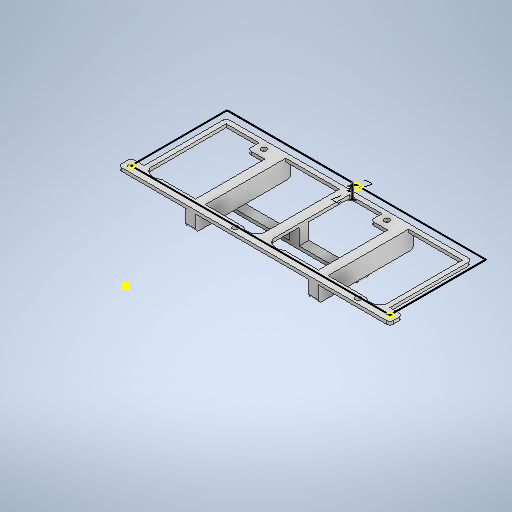
# Autodesk Inventor part: hackatonski skurwiel
Saved by Autodesk Inventor 2025.2 (Build 292293000, 293)
## iProperties
Created: 2026-03-22
Part Number: hackatonski skurwiel
Material: Ogólny
Document SubType Name: Modeling
Designer: janla
Density: 1 g/cm^3
Appearance: Domyślna
Author: janla
Autodesk Inventor part; units mm, degrees
ref_plane "YZ Plane" through (0, 0, 0) normal (1, 0, 0) x (0, 1, 0)
ref_plane "XZ Plane" through (0, 0, 0) normal (0, 1, 0) x (-1, 0, 0)
ref_plane "XY Plane" through (0, 0, 0) normal (0, 0, 1) x (1, 0, 0)
sketch "Szkic1" plane through (0, 0, 0) normal (0, 1, 0) x (-1, 0, 0)
  line L0 (-78.5676, -65.5638) -> (-27.7676, -65.5638)
  line L1 (-27.7676, -65.5638) -> (-27.7676, -111.2838)
  line L2 (-27.7676, -111.2838) -> (-78.5676, -111.2838)
  line L3 (-78.5676, -111.2838) -> (-78.5676, -65.5638)
  circle A0 centre (-78.5676, -65.5638) radius 1.65
  line L4 (-27.7676, -65.5638) -> (-27.7676, -116.3638)
  line L5 (-27.7676, -116.3638) -> (-45.5476, -116.3638)
  circle A1 centre (-45.5476, -116.3638) radius 1.65
  line L6 (-80.2176, -65.5638) -> (-90.2176, -65.5638)
  line L7 (-90.2176, -65.5638) -> (-90.2176, -68.5638)
  line L8 (-90.2176, -68.5638) -> (-90.2176, -62.5638)
  line L9 (-90.2176, -62.5638) -> (-20.2176, -62.5638)
  line L10 (-20.2176, -62.5638) -> (-20.2176, -68.5638)
  line L11 (-20.2176, -68.5638) -> (-90.2176, -68.5638)
  line L12 (-78.5676, -68.5638) -> (-90.2176, -68.5638)
  line L13 (-84.3926, -68.5638) -> (-84.3926, -73.5638)
  circle A2 centre (-84.3926, -73.5638) radius 6.35
  line L14 (-55.2176, -68.5638) -> (-55.2176, -111.2838)
  line L15 (-31.8676, -111.2838) -> (-31.8676, -65.5638)
  line L16 (-20.2176, -65.5638) -> (-20.2176, -68.5638)
  line L17 (-20.2176, -68.5638) -> (-20.2176, -62.5638)
  line L18 (-90.2176, -68.5638) -> (-20.2176, -68.5638)
  line L19 (-31.8676, -68.5638) -> (-20.2176, -68.5638)
  line L20 (-26.0426, -68.5638) -> (-26.0426, -73.5638)
  circle A3 centre (-26.0426, -73.5638) radius 6.35
  line L21 (-45.5476, -116.3638) -> (-40.5476, -116.3638)
  line L22 (-40.5476, -116.3638) -> (-40.5476, -121.3638)
  line L23 (-40.5476, -121.3638) -> (-50.5476, -121.3638)
  line L24 (-50.5476, -121.3638) -> (-50.5476, -111.3638)
  line L25 (-50.5476, -111.3638) -> (-40.5476, -111.3638)
  line L26 (-40.5476, -111.3638) -> (-40.5476, -121.3638)
  line L27 (-45.5476, -116.3638) -> (-54.0476, -116.3638)
  line L28 (-54.0476, -116.3638) -> (-51.0476, -116.3638)
  line L29 (-51.0476, -116.3638) -> (-51.0476, -68.5638)
  line L30 (-51.0476, -68.5638) -> (-54.0476, -68.5638)
  line L31 (-54.0476, -68.5638) -> (-54.0476, -116.3638)
  line L32 (-54.0476, -116.3638) -> (-57.0476, -116.3638)
  line L33 (-57.0476, -116.3638) -> (-57.0476, -68.5638)
  line L34 (-57.0476, -68.5638) -> (-54.0476, -68.5638)
  line L35 (-54.0476, -68.5638) -> (-54.0476, -116.3638)
  line L36 (-57.0476, -116.3638) -> (-50.5476, -116.3638)
  line L37 (-50.5476, -116.3638) -> (-50.5476, -121.3638)
  line L38 (-50.5476, -121.3638) -> (-57.0476, -121.3638)
  line L39 (-57.0476, -121.3638) -> (-57.0476, -116.3638)
  line L40 (-50.5476, -111.3638) -> (-51.0476, -111.3638)
  line L41 (-51.0476, -111.3638) -> (-51.0476, -116.3638)
  line L42 (-51.0476, -116.3638) -> (-50.5476, -116.3638)
  line L43 (-50.5476, -116.3638) -> (-50.5476, -111.3638)
  line L44 (-90.2176, -62.5638) -> (-93.2176, -62.5638)
  line L45 (-93.2176, -62.5638) -> (-93.2176, -68.5638)
  line L46 (-93.2176, -68.5638) -> (-90.2176, -68.5638)
  line L47 (-90.2176, -68.5638) -> (-90.2176, -62.5638)
  line L48 (-57.0476, -121.3638) -> (-93.2176, -121.3638)
  line L49 (-93.2176, -121.3638) -> (-93.2176, -118.3638)
  line L50 (-93.2176, -118.3638) -> (-57.0476, -118.3638)
  line L51 (-57.0476, -118.3638) -> (-57.0476, -121.3638)
  line L52 (-93.2176, -68.5638) -> (-90.2176, -68.5638)
  line L53 (-90.2176, -68.5638) -> (-90.2176, -118.3638)
  line L54 (-90.2176, -118.3638) -> (-93.2176, -118.3638)
  line L55 (-93.2176, -118.3638) -> (-93.2176, -68.5638)
  line L56 (-20.2176, -62.5638) -> (-17.2176, -62.5638)
  line L57 (-17.2176, -62.5638) -> (-17.2176, -68.5638)
  line L58 (-17.2176, -68.5638) -> (-20.2176, -68.5638)
  line L59 (-20.2176, -68.5638) -> (-20.2176, -62.5638)
  line L60 (-17.2176, -68.5638) -> (-20.2176, -68.5638)
  line L61 (-20.2176, -68.5638) -> (-20.2176, -121.3638)
  line L62 (-20.2176, -121.3638) -> (-17.2176, -121.3638)
  line L63 (-17.2176, -121.3638) -> (-17.2176, -68.5638)
  line L64 (-40.5476, -121.3638) -> (-20.2176, -121.3638)
  line L65 (-20.2176, -121.3638) -> (-20.2176, -118.3638)
  line L66 (-20.2176, -118.3638) -> (-40.5476, -118.3638)
  line L67 (-40.5476, -118.3638) -> (-40.5476, -121.3638)
  line L68 (-2.5676, -65.5638) -> (48.2324, -65.5638)
  line L69 (48.2324, -65.5638) -> (48.2324, -111.2838)
  line L70 (48.2324, -111.2838) -> (-2.5676, -111.2838)
  line L71 (-2.5676, -111.2838) -> (-2.5676, -65.5638)
  circle A4 centre (-2.5676, -65.5638) radius 1.65
  line L72 (48.2324, -65.5638) -> (48.2324, -116.3638)
  line L73 (48.2324, -116.3638) -> (30.4524, -116.3638)
  circle A5 centre (30.4524, -116.3638) radius 1.65
  line L74 (-4.2176, -65.5638) -> (-14.2176, -65.5638)
  line L75 (-14.2176, -65.5638) -> (-14.2176, -68.5638)
  line L76 (-14.2176, -68.5638) -> (-14.2176, -62.5638)
  line L77 (-14.2176, -62.5638) -> (55.7824, -62.5638)
  line L78 (55.7824, -62.5638) -> (55.7824, -68.5638)
  line L79 (55.7824, -68.5638) -> (-14.2176, -68.5638)
  line L80 (-2.5676, -68.5638) -> (-14.2176, -68.5638)
  line L81 (-8.3926, -68.5638) -> (-8.3926, -73.5638)
  circle A6 centre (-8.3926, -73.5638) radius 6.35
  line L82 (20.7824, -68.5638) -> (20.7824, -111.2838)
  line L83 (49.9574, -68.5638) -> (49.9574, -73.5638)
  circle A7 centre (49.9574, -73.5638) radius 6.35
  line L84 (44.1324, -68.5638) -> (55.7824, -68.5638)
  line L85 (55.7824, -68.5638) -> (55.7824, -62.5638)
  line L86 (55.7824, -65.5638) -> (55.7824, -68.5638)
  line L87 (44.1324, -111.2838) -> (44.1324, -65.5638)
  line L88 (-14.2176, -68.5638) -> (55.7824, -68.5638)
  line L89 (30.4524, -116.3638) -> (35.4524, -116.3638)
  line L90 (35.4524, -116.3638) -> (35.4524, -121.3638)
  line L91 (35.4524, -121.3638) -> (25.4524, -121.3638)
  line L92 (25.4524, -121.3638) -> (25.4524, -111.3638)
  line L93 (25.4524, -111.3638) -> (35.4524, -111.3638)
  line L94 (35.4524, -111.3638) -> (35.4524, -121.3638)
  line L95 (30.4524, -116.3638) -> (21.9524, -116.3638)
  line L96 (21.9524, -116.3638) -> (24.9524, -116.3638)
  line L97 (24.9524, -116.3638) -> (24.9524, -68.5638)
  line L98 (24.9524, -68.5638) -> (21.9524, -68.5638)
  line L99 (21.9524, -68.5638) -> (21.9524, -116.3638)
  line L100 (21.9524, -116.3638) -> (18.9524, -116.3638)
  line L101 (18.9524, -116.3638) -> (18.9524, -68.5638)
  line L102 (18.9524, -68.5638) -> (21.9524, -68.5638)
  line L103 (21.9524, -68.5638) -> (21.9524, -116.3638)
  line L104 (18.9524, -116.3638) -> (25.4524, -116.3638)
  line L105 (25.4524, -116.3638) -> (25.4524, -121.3638)
  line L106 (25.4524, -121.3638) -> (18.9524, -121.3638)
  line L107 (18.9524, -121.3638) -> (18.9524, -116.3638)
  line L108 (25.4524, -111.3638) -> (24.9524, -111.3638)
  line L109 (24.9524, -111.3638) -> (24.9524, -116.3638)
  line L110 (24.9524, -116.3638) -> (25.4524, -116.3638)
  line L111 (25.4524, -116.3638) -> (25.4524, -111.3638)
  line L112 (-14.2176, -62.5638) -> (-17.2176, -62.5638)
  line L113 (-17.2176, -62.5638) -> (-17.2176, -68.5638)
  line L114 (-17.2176, -68.5638) -> (-14.2176, -68.5638)
  line L115 (-14.2176, -68.5638) -> (-14.2176, -62.5638)
  line L116 (18.9524, -121.3638) -> (-17.2176, -121.3638)
  line L117 (-17.2176, -121.3638) -> (-17.2176, -118.3638)
  line L118 (-17.2176, -118.3638) -> (18.9524, -118.3638)
  line L119 (18.9524, -118.3638) -> (18.9524, -121.3638)
  line L120 (-17.2176, -68.5638) -> (-14.2176, -68.5638)
  line L121 (-14.2176, -68.5638) -> (-14.2176, -118.3638)
  line L122 (-14.2176, -118.3638) -> (-17.2176, -118.3638)
  line L123 (-17.2176, -118.3638) -> (-17.2176, -68.5638)
  line L124 (55.7824, -62.5638) -> (58.7824, -62.5638)
  line L125 (58.7824, -62.5638) -> (58.7824, -68.5638)
  line L126 (58.7824, -68.5638) -> (55.7824, -68.5638)
  line L127 (55.7824, -68.5638) -> (55.7824, -62.5638)
  line L128 (58.7824, -68.5638) -> (55.7824, -68.5638)
  line L129 (55.7824, -68.5638) -> (55.7824, -121.3638)
  line L130 (55.7824, -121.3638) -> (58.7824, -121.3638)
  line L131 (58.7824, -121.3638) -> (58.7824, -68.5638)
  line L132 (35.4524, -121.3638) -> (55.7824, -121.3638)
  line L133 (55.7824, -121.3638) -> (55.7824, -118.3638)
  line L134 (55.7824, -118.3638) -> (35.4524, -118.3638)
  line L135 (35.4524, -118.3638) -> (35.4524, -121.3638)
  point P0 (0, 0)
  point P1 (-90.2176, -71.0356)
  point P2 (-80.4782, -68.5638)
  point P3 (-29.957, -68.5638)
  point P4 (-20.2176, -71.0356)
  point P5 (-14.2176, -71.0356)
  point P6 (-4.4782, -68.5638)
  point P7 (46.043, -68.5638)
  point P8 (55.7824, -71.0356)
  dimension "d2" = 3.3
  dimension "d23" = 3.3
  dimension "d0" = 45.72
  dimension "d1" = 50.8
  dimension "d3" = 50.8
  dimension "d4" = 17.78
  dimension "d5" = 3.3
  dimension "d6" = 10
  dimension "d7" = 3
  dimension "d8" = 6
  dimension "d9" = 70
  dimension "d10" = 5
  dimension "d11" = 5
  dimension "d12" = 5
  dimension "d13" = 10
  dimension "d14" = 10
  dimension "d15" = 8.5
  dimension "d16" = 3
  dimension "d17" = 3
  dimension "d18" = 3
  dimension "d19" = 3
  dimension "d20" = 3
  dimension "d21" = 45.72
  dimension "d22" = 50.8
  dimension "d24" = 50.8
  dimension "d25" = 17.78
  dimension "d26" = 3.3
  dimension "d27" = 10
  dimension "d28" = 3
  dimension "d29" = 6
  dimension "d30" = 70
  dimension "d31" = 5
  dimension "d32" = 5
  dimension "d33" = 5
  dimension "d34" = 10
  dimension "d35" = 10
  dimension "d36" = 8.5
  dimension "d37" = 3
  dimension "d38" = 3
  dimension "d39" = 3
  dimension "d40" = 3
  dimension "d41" = 3
  constraints: 272 end point, 50 parallel, 36 perpendicular, 36 point on line, 28 horizontal, 18 symmetric about line, 8 coincident, 6 centre point, 4 midpoint, 2 horizontal alignment, 2 vertical, 6 other
  measures "d0" distance between parallel lines of L2 L0
  measures "d1" distance between parallel lines of L1 L3
  measures "d3" distance of L0.end L4.end
  measures "d4" distance of L4.end L5.end
  measures "d5" diameter of A1
  measures "d6" distance of L6.start L6.end
  measures "d7" distance of L6.end L7.end
  measures "d8" distance of L7.end L8.end
  measures "d9" distance of L8.end L9.end
  measures "d10" distance of L13.start L13.end
  measures "d11" distance of L21.start L21.end
  measures "d12" distance of L21.end L22.end
  measures "d13" distance of L24.end L25.end
  measures "d14" distance between parallel lines of L25 L23
  measures "d15" distance of L21.start L27.end
  measures "d16" distance of L30.end L29.end
  measures "d17" distance of L33.end L34.end
  measures "d18" distance of L46.end L45.end
  measures "d19" distance between parallel lines of L48 L50
  measures "d20" distance of L57.end L58.end
  measures "d21" distance between parallel lines of L70 L68
  measures "d22" distance between parallel lines of L69 L71
  measures "d24" distance of L68.end L72.end
  measures "d25" distance of L72.end L73.end
  measures "d26" diameter of A5
  measures "d27" distance of L74.start L74.end
  measures "d28" distance of L74.end L75.end
  measures "d29" distance of L75.end L76.end
  measures "d30" distance of L76.end L77.end
  measures "d31" distance of L81.start L81.end
  measures "d32" distance of L89.start L89.end
  measures "d33" distance of L89.end L90.end
  measures "d34" distance of L108.start L93.end
  measures "d35" distance between parallel lines of L93 L91
  measures "d36" distance of L89.start L103.end
  measures "d37" distance of L98.end L98.start
  measures "d38" distance of L101.end L103.start
  measures "d39" distance of L114.end L123.end
  measures "d40" distance between parallel lines of L116 L118
  measures "d41" distance of L131.end L126.end
extrude "Wyciągnięcie proste1" add sketch "Szkic1" along normal blind 2 contours A0 L6 L8 L9 L10 L11 A3 L1 L0 | L0 L15 L11 L3 A0 | L3 L11 A2 L7 L6 A0 | L0 L1 A3 L11 L15 | L7 L46 L45 L44 L8 | L11 L14 L2 L33 | L29 L2 L31 L11 | L53 A2 L50 L55 L46 | L11 A2 L53 | L11 L31 L2 L14 | L2 L31 L32 L33 | L11 L61 A3 | L29 L27 L31 L2 | L53 A2 | L56 L57 L58 L10 | L32 L27 L24 L38 L39 | L58 L63 L62 L61 A3 | A3 L61 | L40 L24 L27 L29 | L50 L39 L48 L49 | L112 L76 L75 L114 L57 | L114 L121 A6 L118 L63 | L25 L26 L5 A1 L27 L24 | L77 L78 L79 A7 L69 L68 A4 L74 L76 | L61 L64 L22 L66 | L118 L107 L116 L63 | L75 L74 A4 L71 L79 A6 | L79 A6 L121 | L27 A1 L5 L22 L23 L24 | L124 L125 L126 L78 | L121 A6 | L107 L100 L95 L92 L106 | L68 L87 L79 L71 A4 | L129 A7 L79 | L126 L131 L130 L129 A7 | L92 L95 A5 L73 L90 L91 | L101 L70 L99 L100 | L68 L69 A7 L79 L87 | A7 L129 | L90 L134 L129 L132 | L95 L97 L108 L92 | L92 L93 L94 L73 A5 L95 | L99 L70 L97 L95 | L101 L79 L82 L70 | L99 L79 L97 L70 | L70 L82 L79 L99
sketch "Szkic2" plane through (0, 0, 0) normal (0, -1, 0) x (1, 0, 0)
  line L0 (-24.9524, -111.3638) -> (-24.9524, -68.5638) projected
  line L1 (-18.9524, -68.5638) -> (-18.9524, -118.3638) projected
  line L2 (-24.9524, -68.5638) -> (-18.9524, -68.5638)
  line L3 (-18.9524, -68.5638) -> (-18.9524, -118.3638)
  line L4 (-18.9524, -118.3638) -> (-24.9524, -118.3638)
  line L5 (-24.9524, -118.3638) -> (-24.9524, -68.5638)
  line L6 (93.2176, -121.3638) -> (-58.7824, -121.3638) projected
  line L7 (-18.9524, -118.3638) -> (-24.9524, -118.3638)
  line L8 (-24.9524, -118.3638) -> (-24.9524, -121.3638)
  line L9 (-24.9524, -121.3638) -> (-18.9524, -121.3638)
  line L10 (-18.9524, -121.3638) -> (-18.9524, -118.3638)
  line L11 (-58.7824, -62.5638) -> (93.2176, -62.5638) projected
  line L12 (-24.9524, -68.5638) -> (-18.9524, -68.5638)
  line L13 (-18.9524, -68.5638) -> (-18.9524, -62.5638)
  line L14 (-18.9524, -62.5638) -> (-24.9524, -62.5638)
  line L15 (-24.9524, -62.5638) -> (-24.9524, -68.5638)
  line L16 (57.0476, -68.5638) -> (57.0476, -118.3638) projected
  line L17 (51.0476, -111.3638) -> (51.0476, -68.5638) projected
  line L18 (57.0476, -118.3638) -> (51.0476, -118.3638)
  line L19 (51.0476, -118.3638) -> (51.0476, -68.5638)
  line L20 (51.0476, -68.5638) -> (57.0476, -68.5638)
  line L21 (57.0476, -68.5638) -> (57.0476, -118.3638)
  line L22 (51.0476, -68.5638) -> (57.0476, -68.5638)
  line L23 (57.0476, -68.5638) -> (57.0476, -62.5638)
  line L24 (57.0476, -62.5638) -> (51.0476, -62.5638)
  line L25 (51.0476, -62.5638) -> (51.0476, -68.5638)
  line L26 (51.0476, -118.3638) -> (57.0476, -118.3638)
  line L27 (57.0476, -118.3638) -> (57.0476, -121.3638)
  line L28 (57.0476, -121.3638) -> (51.0476, -121.3638)
  line L29 (51.0476, -121.3638) -> (51.0476, -118.3638)
  point P0 (0, 0)
  constraints: 48 end point, 12 parallel, 8 point on line, 6 horizontal, 6 perpendicular
extrude "Wyciągnięcie proste2" add sketch "Szkic2" along normal blind 10 contours L0 L2 L1 L4 L5 | L15 L11 L13 L2 | L4 L10 L6 L8 | L11 L23 L20 L25 | L29 L18 L27 L6 | L20 L16 L18 L19 L17
sketch "Szkic4" plane through (0, -10, 0) normal (0, -1, 0) x (1, 0, 0)
  line L0 (57.0476, -68.5638) -> (57.0476, -118.3638) projected
  line L1 (-24.9524, -111.3638) -> (-24.9524, -68.5638) projected
  line L2 (57.0476, -93.4638) -> (-24.9524, -93.4638)
  line L3 (-24.9524, -93.4638) -> (-24.9524, -87.4638)
  line L4 (-24.9524, -87.4638) -> (57.0476, -87.4638)
  line L5 (57.0476, -87.4638) -> (57.0476, -93.4638)
  point P0 (0, 0)
  point P1 (57.0476, -87.4638)
  point P2 (-24.9524, -93.4638)
  dimension "d47" = 6
  constraints: 8 end point, 2 parallel, 1 horizontal, 1 midpoint, 1 perpendicular, 1 point on line
  measures "d47" distance between parallel lines of L2 L4
extrude "Wyciągnięcie proste3" add sketch "Szkic4" along normal blind 2
sketch "Szkic5" plane through (0, -10, 0) normal (0, 1, 0) x (1, 0, 0)
  line L0 (20.2176, 71.0356) -> (20.2176, 118.3638) projected
  line L1 (20.2176, 93.2735) -> (20.2176, 93.4638)
  line L2 (-18.9524, 93.4638) -> (51.0476, 93.4638) projected
  line L3 (20.2176, 93.4638) -> (13.4187, 87.4638)
  line L4 (51.0476, 87.4638) -> (-18.9524, 87.4638) projected
  line L5 (13.4187, 87.4638) -> (14.2176, 87.4638)
  line L6 (14.2176, 118.3638) -> (14.2176, 71.0356) projected
  line L7 (14.2176, 87.4638) -> (20.2176, 87.4638)
  line L8 (20.2176, 87.4638) -> (20.2176, 93.4638)
  line L9 (20.2176, 93.4638) -> (14.2176, 93.4638)
  line L10 (14.2176, 93.4638) -> (14.2176, 87.4638)
  point P0 (0, 0)
  point P1 (14.2176, 93.4638)
  point P2 (20.2176, 87.4638)
  constraints: 14 end point, 4 point on line, 2 parallel, 2 perpendicular, 1 horizontal, 1 vertical
extrude "Wyciągnięcie proste4" add sketch "Szkic5" along normal blind 10 contours L4 L6 L3 L0 | L3 L6 L2
sketch "Szkic6" plane through (51.0476, 0, -121.3638) normal (0, 0, -1) x (-1, 0, 0)
  line L0 (30.83, -10) -> (30.83, 0) projected
  line L1 (36.83, 0) -> (36.83, 2) projected
  line L2 (30.83, 0) -> (36.83, 0)
  line L3 (36.83, 0) -> (36.83, 2)
  line L4 (36.83, 2) -> (30.83, 2)
  line L5 (30.83, 2) -> (30.83, 0)
  point P0 (51.0476, 0)
  constraints: 8 end point, 2 parallel, 1 horizontal, 1 perpendicular
extrude "Wyciągnięcie proste5" add sketch "Szkic6" along normal blind 8
sketch "Szkic7" plane through (-58.7824, 0, -121.3638) normal (-1, 0, 0) x (0, 0, 1)
  line L0 (58.8, 0) -> (58.8, 2) projected
  line L1 (50.3282, 0) -> (54.15, 0) projected
  line L2 (58.8, 2) -> (50.8, 2)
  line L3 (50.8, 2) -> (50.8, 0)
  line L4 (50.8, 0) -> (58.8, 0)
  line L5 (58.8, 0) -> (58.8, 2)
  point P0 (121.3638, 0)
  point P1 (52.8, 0)
  dimension "d54" = 8
  constraints: 8 end point, 2 parallel, 1 horizontal, 1 perpendicular, 1 point on line
  measures "d54" distance of L4.end L3.end
extrude "Wyciągnięcie proste6" add sketch "Szkic7" along normal blind 8
sketch "Szkic8" plane through (93.2176, 0, -62.5638) normal (1, 0, 0) x (0, 0, -1)
  line L0 (0, 0) -> (0, 2) projected
  line L1 (0, 2) -> (8, 2)
  line L2 (8, 2) -> (8, 0)
  line L3 (8, 0) -> (0, 0)
  line L4 (0, 0) -> (0, 2)
  point P0 (-62.5638, 0)
  dimension "d57" = 8
  constraints: 8 end point, 2 parallel, 1 horizontal, 1 perpendicular
  measures "d57" distance of L2.end L3.end
extrude "Wyciągnięcie proste7" add sketch "Szkic8" along normal blind 8
sketch "Szkic9" plane through (0, 2, 0) normal (0, 1, 0) x (1, 0, 0)
  line L0 (-24.9524, 62.5638) -> (-66.7824, 62.5638) projected
  line L1 (-58.7824, 70.5638) -> (-66.7824, 70.5638) projected
  line L2 (-66.7824, 62.5638) -> (-58.7824, 70.5638)
  line L3 (-58.7824, 70.5638) -> (-66.7824, 70.5638)
  line L4 (-66.7824, 70.5638) -> (-58.7824, 62.5638)
  circle A0 centre (-62.7824, 66.5638) radius 1.65
  line L5 (20.2176, 93.4638) -> (14.2176, 93.4638) projected
  line L6 (17.2176, 93.4638) -> (17.2176, 62.5638)
  line L7 (-18.9524, 62.5638) -> (51.0476, 62.5638) projected
  line L8 (93.2176, 70.5638) -> (101.2176, 70.5638)
  line L9 (101.2176, 62.5638) -> (93.2176, 70.5638)
  line L10 (93.2176, 70.5638) -> (101.2176, 70.5638)
  line L11 (101.2176, 70.5638) -> (93.2176, 62.5638)
  circle A1 centre (97.2176, 66.5638) radius 1.65
  line L12 (14.2176, 121.3638) -> (14.2176, 129.3638) projected
  line L13 (93.2176, 121.3638) -> (20.2176, 121.3638) projected
  line L14 (14.2176, 129.3638) -> (20.2176, 121.3638)
  line L15 (20.2176, 121.3638) -> (20.2176, 129.3638)
  line L16 (20.2176, 129.3638) -> (14.2176, 121.3638)
  line L17 (17.2176, 125.3638) -> (17.2176, 125.8638)
  circle A2 centre (17.2176, 125.8638) radius 1.65
  point P0 (0, 0)
  dimension "d60" = 3.3
  dimension "d61" = 0.5
  dimension "d62" = 3.3
  constraints: 24 end point, 5 symmetric about line, 3 centre point, 3 midpoint, 2 perpendicular, 2 vertical, 1 coincident, 1 collinear, 1 point on line, 1 other
  measures "d60" diameter of A0
  measures "d61" distance of L17.start L17.end
  measures "d62" diameter of A2
extrude "Wyciągnięcie proste8" cut sketch "Szkic9" against normal blind 8 contours A0 L2 L4 | L4 L2 A0 | A0 L4 L2 | L4 A0 L2 | A1 L11 L9 | L9 L11 A1 | A1 L9 L11 | L9 A1 L11 | A2 L14 L16 | L16 L14 A2 | A2 L16 L14 | L16 A2 L14
fillet "Zaokrąglenie1" radius 2 16 edges at (101.2176, 1, -70.5638) (101.2176, 1, -62.5638) (-66.7824, 1, -62.5638) (-66.7824, 1, -70.5638) (-58.7824, 1, -121.3638) (-35.4524, 1, -111.3638) (40.5476, 1, -111.3638) (20.2176, 1, -129.3638) (14.2176, 1, -129.3638) (54.0476, -10, -121.3638) (54.0476, -10, -62.5638) (-21.9524, -10, -62.5638) (-21.9524, -10, -121.3638) (93.2176, 1, -121.3638) (57.0476, -12, -90.4638) (-24.9524, -12, -90.4638)
sketch "Szkic10" plane through (0, 2, 0) normal (0, 1, 0) x (1, 0, 0)
  circle A0 centre (97.2176, 66.5638) radius 1.65 projected
  circle A1 centre (-62.7824, 66.5638) radius 1.65 projected
  line L0 (97.2176, 66.5638) -> (-62.7824, 66.5638)
  circle A2 centre (17.2176, 125.8638) radius 1.65 projected
  line L1 (17.2176, 125.8638) -> (-62.7824, 125.8638)
  line L2 (-62.7824, 125.8638) -> (97.2176, 125.8638)
  line L3 (97.2176, 125.8638) -> (97.2176, 66.5638)
  line L4 (-62.7824, 66.5638) -> (-62.7824, 125.8638)
  line L5 (97.2176, 125.8638) -> (97.2176, 66.5638)
  line L6 (20.2176, 121.3638) -> (20.2176, 127.3638) projected
  line L7 (20.2176, 121.3638) -> (20.2176, 120.3638)
  line L8 (20.2176, 120.3638) -> (17.2176, 120.3638)
  line L9 (17.2176, 120.3638) -> (17.2176, 125.8638)
  point P0 (0, 0)
  dimension "d66" = 1
  constraints: 18 end point, 4 perpendicular, 2 horizontal, 1 parallel, 1 point on line, 1 vertical
  measures "d66" distance of L6.start L7.end
sketch "Szkic11" plane through (0, 2, 0) normal (0, 1, 0) x (1, 0, 0)
  line L0 (14.2176, 121.3638) -> (14.2176, 127.3638) projected
  line L1 (14.2176, 121.3638) -> (24.1883, 121.3638)
  line L2 (24.1883, 121.3638) -> (24.1883, 131.5439)
  line L3 (24.1883, 131.5439) -> (14.2176, 131.5439)
  line L4 (14.2176, 131.5439) -> (14.2176, 121.3638)
  point P0 (0, 0)
  constraints: 8 end point, 2 parallel, 1 horizontal, 1 perpendicular
extrude "Wyciągnięcie proste9" cut sketch "Szkic11" against normal blind 8
